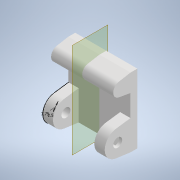
# Autodesk Inventor part: Encoder_Mount1_Slider
Saved by Autodesk Inventor 2022 (Build 260153000, 153)
## iProperties
Created: 2024-04-26
Part Number: Encoder_Mount1_Slider
Material: Generic
Document SubType Name: Modeling
Designer: raphael.hauk
Density: 1 g/cm^3
Appearance: Default
Author: raphael.hauk
Autodesk Inventor part; units mm, degrees
ref_plane "YZ Plane" through (0, 0, 0) normal (1, 0, 0) x (0, 1, 0)
ref_plane "XZ Plane" through (0, 0, 0) normal (0, 1, 0) x (-1, 0, 0)
ref_plane "XY Plane" through (0, 0, 0) normal (0, 0, 1) x (1, 0, 0)
sketch "Sketch1" plane through (0, 0, 0) normal (0, 0, 1) x (1, 0, 0)
  line L0 (2.0907, -12.7904) -> (2.0907, 12.2096)
  line L1 (2.0907, 12.2096) -> (-15.9093, 12.2096)
  line L2 (-15.9093, 12.2096) -> (-15.9093, -12.7904)
  line L3 (-15.9093, -12.7904) -> (2.0907, -12.7904) projected
  line L4 (-15.9093, 17.2096) -> (-15.9093, -14.7904) construction
  line L5 (2.0907, -14.7904) -> (2.0907, 17.2096) construction
  dimension "d27" = 25
  constraints: 6 end point, 2 point on line
  measures "d27" distance between parallel lines of L3 L1
extrude "Extrusion1" add sketch "Sketch1" along normal blind 2
sketch "Sketch2" plane through (-15.9093, -7.7904, 0) normal (-1, 0, 0) x (0, 0, 1)
  circle A0 centre (5.7, -0.7) radius 1.25 construction
  line L0 (2, -5) -> (6.216, -4.4143)
  arc A1 (6.216, -4.4143) -> (6.216, 3.0143) centre (5.7, -0.7) ccw
  line L1 (5.7, -0.7) -> (2, -0.7) construction
  line L2 (2, 3.6) -> (6.216, 3.0143)
  line L3 (2, 3.6) -> (2, -5)
  line L4 (0, -5) -> (2, -5) construction
  arc A2 (4.4, -0.7) -> (7, -0.7) centre (5.7, -0.7) ccw construction
  dimension "d2" = 2.5
  dimension "d3" = 3.75
  constraints: 8 end point, 4 point on circle, 3 centre point, 3 coincident, 2 symmetric about line, 1 horizontal, 1 tangent, 1 vertical, 4 other
  measures "d2" diameter of A0
  measures "d3" radius of A1
extrude "Extrusion2" add sketch "Sketch2" against normal blind 3
ref_plane "Work Plane1" through (-6.9093, -12.7904, 0) normal (-1, 0, 0) x (0, 0, 1)
mirror "Mirror1" about plane through (-6.9093, -12.7904, 0) normal (-1, 0, 0) of "Extrusion2"
hole "Hole1" at (-15.9093, -8.4904, 5.7) direction (1, 0, 0) diameter 2.6 end through all clearance for "Socket Head Cap Screw ISO 4762" size "M2.5" standard "ISO"
sketch "Sketch3" plane through (-0.9093, -8.4904, 5.7) normal (-1, 0, 0) x (0, 0, 1)
  circle A0 centre (0, 0) radius 1.3 projected
  line L0 (-1.4722, -2.55) -> (-2.9445, 0)
  line L1 (-2.9445, 0) -> (-1.4722, 2.55)
  line L2 (-1.4722, 2.55) -> (1.4722, 2.55)
  line L3 (1.4722, 2.55) -> (2.9445, 0)
  line L4 (2.9445, 0) -> (1.4722, -2.55)
  line L5 (1.4722, -2.55) -> (-1.4722, -2.55)
  point P0 (-5.7, 8.4904)
  point P1 (0, 0)
  dimension "d18" = 5.1
  constraints: 12 end point, 1 coincident, 1 horizontal, 13 other
  measures "d18" distance between parallel lines of L5 L2
extrude "Extrusion3" cut sketch "Sketch3" against normal blind 2.1
sketch "Sketch4" plane through (-15.9093, -12.7904, 0) normal (-1, 0, 0) x (0, 0, 1)
  arc A0 (5.3473, 20.4706) -> (5.3473, 24.4098) centre (5, 22.4402) ccw
  line L0 (5, 22.4402) -> (2, 22.4402) construction
  line L1 (2, 25) -> (2, 8.6) construction
  line L2 (5.3473, 24.4098) -> (2, 25)
  line L3 (5.3473, 20.4706) -> (2, 19.8803)
  line L4 (2, 25) -> (2, 19.8803)
  point P0 (0, 12.7904)
  dimension "d21" = 2
  dimension "d22" = 3
  dimension "d24" = 80
  constraints: 8 end point, 2 point on circle, 2 symmetric about line, 1 centre point, 1 horizontal, 1 point on line, 1 tangent, 1 vertical
  measures "d21" radius of A0
  measures "d22" distance of L0.start L0.end
  measures "d24" angle of L1 L2
extrude "Extrusion4" add sketch "Sketch4" against normal up to surface (18 mm away)
thicken "Thicken1" operation add thickness 0.1 both sides no extend neighbours yes toward (-1, 0, 0) faces at (2.0907, -1.5904, 0.6667)
thicken "Thicken2" operation add thickness 0.1 both sides no extend neighbours yes toward (0, 0, 1) faces at (-3.976, -4.4571, 0)
body "Solid1"
